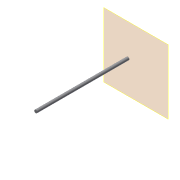
# Autodesk Inventor part: ServoHolderPole
Saved by Autodesk Inventor 2018 (Build 220112000, 112)
## iProperties
Created: 2018-10-17
Part Number: ServoHolderPole
Material: Generic
Document SubType Name: Modeling
Designer: Vulnic
Density: 1 g/cm^3
Appearance: Default
Author: Vulnic
Autodesk Inventor part; units mm, degrees
ref_plane "YZ Plane" through (0, 0, 0) normal (1, 0, 0) x (0, 1, 0)
ref_plane "XZ Plane" through (0, 0, 0) normal (0, 1, 0) x (-1, 0, 0)
ref_plane "XY Plane" through (0, 0, 0) normal (0, 0, 1) x (1, 0, 0)
ref_plane "Work Plane1" through (-24.2528, 17.7674, 5.1586) normal (0, 0, 1) x (1, 0.0008, 0)
sketch "Sketch1" plane through (-24.2528, 17.7674, 5.1586) normal (0, 0, 1) x (1, 0.0008, 0)
  circle A0 centre (-4.87, 0.1884) radius 0.9
  circle A1 centre (-4.87, 0.1884) radius 0.9
  point P0 (24.238, -17.7876)
  dimension "d1" = 1.8
  constraints: 2 centre point, 1 coincident, 1 concentric
  measures "d1" diameter of A0
extrude "Extrusion1" add sketch "Sketch1" along normal blind 55
body "Solid1"
